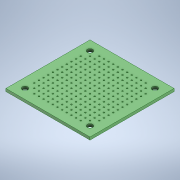
# Autodesk Inventor part: PCB
Saved by Autodesk Inventor 2020.5 (Build 245400000, 400)
## iProperties
Created: 2022-12-14
Part Number: PCB
Material: Generic
Document SubType Name: Modeling
Designer: aivel
Density: 1 g/cm^3
Appearance: Smooth - Dark Forest Green
Author: aivel
Autodesk Inventor part; units mm, degrees
ref_plane "YZ Plane" through (0, 0, 0) normal (1, 0, 0) x (0, 1, 0)
ref_plane "XZ Plane" through (0, 0, 0) normal (0, 1, 0) x (-1, 0, 0)
ref_plane "XY Plane" through (0, 0, 0) normal (0, 0, 1) x (1, 0, 0)
sketch "Sketch1" plane through (0, 0, 0) normal (0, 1, 0) x (-1, 0, 0)
  line L0 (0, 0) -> (-46, 0)
  line L1 (-46, 0) -> (-46, -46)
  line L2 (-46, -46) -> (0, -46)
  line L3 (0, -46) -> (0, 0)
  circle A0 centre (-23, -23) radius 0.375
  line L4 (-23, -46) -> (-23, 0) construction
  line L5 (-46, -23) -> (0, -23) construction
  circle A1 centre (-25.54, -23) radius 0.375
  circle A2 centre (-28.08, -23) radius 0.375
  circle A3 centre (-30.62, -23) radius 0.375
  circle A4 centre (-33.16, -23) radius 0.375
  circle A5 centre (-35.7, -23) radius 0.375
  circle A6 centre (-38.24, -23) radius 0.375
  circle A7 centre (-40.78, -23) radius 0.375
  circle A8 centre (-23, -20.46) radius 0.375
  circle A9 centre (-23, -17.92) radius 0.375
  circle A10 centre (-23, -15.38) radius 0.375
  circle A11 centre (-23, -12.84) radius 0.375
  circle A12 centre (-23, -10.3) radius 0.375
  circle A13 centre (-23, -7.76) radius 0.375
  circle A14 centre (-23, -5.22) radius 0.375
  circle A15 centre (-20.46, -20.46) radius 0.375
  circle A16 centre (-20.46, -17.92) radius 0.375
  circle A17 centre (-20.46, -15.38) radius 0.375
  circle A18 centre (-20.46, -12.84) radius 0.375
  circle A19 centre (-20.46, -10.3) radius 0.375
  circle A20 centre (-20.46, -7.76) radius 0.375
  circle A21 centre (-20.46, -5.22) radius 0.375
  circle A22 centre (-17.92, -20.46) radius 0.375
  circle A23 centre (-17.92, -17.92) radius 0.375
  circle A24 centre (-17.92, -15.38) radius 0.375
  circle A25 centre (-17.92, -12.84) radius 0.375
  circle A26 centre (-17.92, -10.3) radius 0.375
  circle A27 centre (-17.92, -7.76) radius 0.375
  circle A28 centre (-17.92, -5.22) radius 0.375
  circle A29 centre (-15.38, -20.46) radius 0.375
  circle A30 centre (-15.38, -17.92) radius 0.375
  circle A31 centre (-15.38, -15.38) radius 0.375
  circle A32 centre (-15.38, -12.84) radius 0.375
  circle A33 centre (-15.38, -10.3) radius 0.375
  circle A34 centre (-15.38, -7.76) radius 0.375
  circle A35 centre (-15.38, -5.22) radius 0.375
  circle A36 centre (-12.84, -20.46) radius 0.375
  circle A37 centre (-12.84, -17.92) radius 0.375
  circle A38 centre (-12.84, -15.38) radius 0.375
  circle A39 centre (-12.84, -12.84) radius 0.375
  circle A40 centre (-12.84, -10.3) radius 0.375
  circle A41 centre (-12.84, -7.76) radius 0.375
  circle A42 centre (-12.84, -5.22) radius 0.375
  circle A43 centre (-10.3, -20.46) radius 0.375
  circle A44 centre (-10.3, -17.92) radius 0.375
  circle A45 centre (-10.3, -15.38) radius 0.375
  circle A46 centre (-10.3, -12.84) radius 0.375
  circle A47 centre (-10.3, -10.3) radius 0.375
  circle A48 centre (-10.3, -7.76) radius 0.375
  circle A49 centre (-10.3, -5.22) radius 0.375
  circle A50 centre (-7.76, -20.46) radius 0.375
  circle A51 centre (-7.76, -17.92) radius 0.375
  circle A52 centre (-7.76, -15.38) radius 0.375
  circle A53 centre (-7.76, -12.84) radius 0.375
  circle A54 centre (-7.76, -10.3) radius 0.375
  circle A55 centre (-7.76, -7.76) radius 0.375
  circle A56 centre (-5.22, -20.46) radius 0.375
  circle A57 centre (-5.22, -17.92) radius 0.375
  circle A58 centre (-5.22, -15.38) radius 0.375
  circle A59 centre (-5.22, -12.84) radius 0.375
  circle A60 centre (-5.22, -10.3) radius 0.375
  circle A61 centre (-35.7, -23) radius 0.375
  circle A62 centre (-33.16, -23) radius 0.375
  circle A63 centre (-35.7, -20.46) radius 0.375
  circle A64 centre (-33.16, -20.46) radius 0.375
  circle A65 centre (-30.62, -23) radius 0.375
  circle A66 centre (-35.7, -17.92) radius 0.375
  circle A67 centre (-30.62, -17.92) radius 0.375
  circle A68 centre (-28.08, -23) radius 0.375
  circle A69 centre (-25.54, -20.46) radius 0.375
  circle A70 centre (-25.54, -17.92) radius 0.375
  circle A71 centre (-23, -20.46) radius 0.375
  circle A72 centre (-23, -17.92) radius 0.375
  circle A73 centre (-23, -15.38) radius 0.375
  circle A74 centre (-28.08, -17.92) radius 0.375
  circle A75 centre (-30.62, -20.46) radius 0.375
  circle A76 centre (-25.54, -23) radius 0.375
  circle A77 centre (-28.08, -20.46) radius 0.375
  circle A78 centre (-23, -12.84) radius 0.375
  circle A79 centre (-23, -10.3) radius 0.375
  circle A80 centre (-30.62, -15.38) radius 0.375
  circle A81 centre (-23, -7.76) radius 0.375
  circle A82 centre (-23, -5.22) radius 0.375
  circle A83 centre (-25.54, -15.38) radius 0.375
  circle A84 centre (-28.08, -12.84) radius 0.375
  circle A85 centre (-28.08, -15.38) radius 0.375
  circle A86 centre (-25.54, -12.84) radius 0.375
  circle A87 centre (-30.62, -12.84) radius 0.375
  circle A88 centre (-25.54, -10.3) radius 0.375
  circle A89 centre (-25.54, -7.76) radius 0.375
  circle A90 centre (-25.54, -5.22) radius 0.375
  circle A91 centre (-33.16, -12.84) radius 0.375
  circle A92 centre (-33.16, -17.92) radius 0.375
  circle A93 centre (-35.7, -15.38) radius 0.375
  circle A94 centre (-33.16, -15.38) radius 0.375
  circle A95 centre (-35.7, -12.84) radius 0.375
  circle A96 centre (-28.08, -10.3) radius 0.375
  circle A97 centre (-28.08, -7.76) radius 0.375
  circle A98 centre (-28.08, -5.22) radius 0.375
  circle A99 centre (-30.62, -10.3) radius 0.375
  circle A100 centre (-30.62, -7.76) radius 0.375
  circle A101 centre (-30.62, -5.22) radius 0.375
  circle A102 centre (-35.7, -10.3) radius 0.375
  circle A103 centre (-33.16, -7.76) radius 0.375
  circle A104 centre (-35.7, -7.76) radius 0.375
  circle A105 centre (-33.16, -5.22) radius 0.375
  circle A106 centre (-35.7, -5.22) radius 0.375
  circle A107 centre (-33.16, -10.3) radius 0.375
  circle A108 centre (-38.24, -12.84) radius 0.375
  circle A109 centre (-40.78, -12.84) radius 0.375
  circle A110 centre (-40.78, -10.3) radius 0.375
  circle A111 centre (-38.24, -7.76) radius 0.375
  circle A112 centre (-38.24, -10.3) radius 0.375
  circle A113 centre (-38.24, -15.38) radius 0.375
  circle A114 centre (-40.78, -15.38) radius 0.375
  circle A115 centre (-38.24, -17.92) radius 0.375
  circle A116 centre (-40.78, -17.92) radius 0.375
  circle A117 centre (-38.24, -20.46) radius 0.375
  circle A118 centre (-40.78, -20.46) radius 0.375
  circle A119 centre (-38.24, -23) radius 0.375
  circle A120 centre (-40.78, -23) radius 0.375
  circle A121 centre (-10.3, -23) radius 0.375
  circle A122 centre (-12.84, -23) radius 0.375
  circle A123 centre (-15.38, -23) radius 0.375
  circle A124 centre (-17.92, -23) radius 0.375
  circle A125 centre (-20.46, -23) radius 0.375
  circle A126 centre (-7.76, -23) radius 0.375
  circle A127 centre (-5.22, -23) radius 0.375
  circle A128 centre (-17.92, -23) radius 0.375
  circle A129 centre (-15.38, -23) radius 0.375
  circle A130 centre (-12.84, -23) radius 0.375
  circle A131 centre (-10.3, -23) radius 0.375
  circle A132 centre (-7.76, -23) radius 0.375
  circle A133 centre (-5.22, -23) radius 0.375
  circle A134 centre (-20.46, -23) radius 0.375
  circle A135 centre (-25.54, -38.24) radius 0.375
  circle A136 centre (-23, -38.24) radius 0.375
  circle A137 centre (-23, -38.24) radius 0.375
  circle A138 centre (-25.54, -35.7) radius 0.375
  circle A139 centre (-23, -35.7) radius 0.375
  circle A140 centre (-28.08, -35.7) radius 0.375
  circle A141 centre (-23, -40.78) radius 0.375
  circle A142 centre (-23, -40.78) radius 0.375
  circle A143 centre (-28.08, -40.78) radius 0.375
  circle A144 centre (-23, -35.7) radius 0.375
  circle A145 centre (-25.54, -40.78) radius 0.375
  circle A146 centre (-28.08, -38.24) radius 0.375
  circle A147 centre (-23, -33.16) radius 0.375
  circle A148 centre (-23, -33.16) radius 0.375
  circle A149 centre (-23, -30.62) radius 0.375
  circle A150 centre (-23, -30.62) radius 0.375
  circle A151 centre (-23, -28.08) radius 0.375
  circle A152 centre (-23, -28.08) radius 0.375
  circle A153 centre (-23, -25.54) radius 0.375
  circle A154 centre (-25.54, -33.16) radius 0.375
  circle A155 centre (-25.54, -30.62) radius 0.375
  circle A156 centre (-28.08, -33.16) radius 0.375
  circle A157 centre (-28.08, -30.62) radius 0.375
  circle A158 centre (-30.62, -30.62) radius 0.375
  circle A159 centre (-23, -25.54) radius 0.375
  circle A160 centre (-20.46, -25.54) radius 0.375
  circle A161 centre (-20.46, -28.08) radius 0.375
  circle A162 centre (-28.08, -25.54) radius 0.375
  circle A163 centre (-28.08, -28.08) radius 0.375
  circle A164 centre (-25.54, -28.08) radius 0.375
  circle A165 centre (-20.46, -30.62) radius 0.375
  circle A166 centre (-17.92, -25.54) radius 0.375
  circle A167 centre (-15.38, -25.54) radius 0.375
  circle A168 centre (-12.84, -25.54) radius 0.375
  circle A169 centre (-20.46, -33.16) radius 0.375
  circle A170 centre (-20.46, -35.7) radius 0.375
  circle A171 centre (-20.46, -38.24) radius 0.375
  circle A172 centre (-20.46, -40.78) radius 0.375
  circle A173 centre (-17.92, -33.16) radius 0.375
  circle A174 centre (-17.92, -35.7) radius 0.375
  circle A175 centre (-17.92, -38.24) radius 0.375
  circle A176 centre (-17.92, -40.78) radius 0.375
  circle A177 centre (-15.38, -33.16) radius 0.375
  circle A178 centre (-15.38, -35.7) radius 0.375
  circle A179 centre (-15.38, -38.24) radius 0.375
  circle A180 centre (-15.38, -40.78) radius 0.375
  circle A181 centre (-12.84, -33.16) radius 0.375
  circle A182 centre (-12.84, -38.24) radius 0.375
  circle A183 centre (-12.84, -40.78) radius 0.375
  circle A184 centre (-12.84, -35.7) radius 0.375
  circle A185 centre (-17.92, -28.08) radius 0.375
  circle A186 centre (-17.92, -30.62) radius 0.375
  circle A187 centre (-15.38, -28.08) radius 0.375
  circle A188 centre (-15.38, -30.62) radius 0.375
  circle A189 centre (-12.84, -28.08) radius 0.375
  circle A190 centre (-12.84, -30.62) radius 0.375
  circle A191 centre (-10.3, -25.54) radius 0.375
  circle A192 centre (-10.3, -28.08) radius 0.375
  circle A193 centre (-10.3, -30.62) radius 0.375
  circle A194 centre (-10.3, -35.7) radius 0.375
  circle A195 centre (-10.3, -38.24) radius 0.375
  circle A196 centre (-10.3, -40.78) radius 0.375
  circle A197 centre (-10.3, -33.16) radius 0.375
  circle A198 centre (-7.76, -35.7) radius 0.375
  circle A199 centre (-7.76, -38.24) radius 0.375
  circle A200 centre (-7.76, -33.16) radius 0.375
  circle A201 centre (-5.22, -35.7) radius 0.375
  circle A202 centre (-5.22, -33.16) radius 0.375
  circle A203 centre (-7.76, -30.62) radius 0.375
  circle A204 centre (-5.22, -30.62) radius 0.375
  circle A205 centre (-7.76, -28.08) radius 0.375
  circle A206 centre (-5.22, -28.08) radius 0.375
  circle A207 centre (-7.76, -25.54) radius 0.375
  circle A208 centre (-5.22, -25.54) radius 0.375
  circle A209 centre (-33.16, -30.62) radius 0.375
  circle A210 centre (-35.7, -30.62) radius 0.375
  circle A211 centre (-30.62, -25.54) radius 0.375
  circle A212 centre (-30.62, -28.08) radius 0.375
  circle A213 centre (-33.16, -28.08) radius 0.375
  circle A214 centre (-35.7, -28.08) radius 0.375
  circle A215 centre (-35.7, -25.54) radius 0.375
  circle A216 centre (-33.16, -25.54) radius 0.375
  circle A217 centre (-38.24, -30.62) radius 0.375
  circle A218 centre (-38.24, -28.08) radius 0.375
  circle A219 centre (-38.24, -25.54) radius 0.375
  circle A220 centre (-40.78, -30.62) radius 0.375
  circle A221 centre (-40.78, -28.08) radius 0.375
  circle A222 centre (-40.78, -25.54) radius 0.375
  circle A223 centre (-30.62, -33.16) radius 0.375
  circle A224 centre (-30.62, -35.7) radius 0.375
  circle A225 centre (-30.62, -38.24) radius 0.375
  circle A226 centre (-33.16, -33.16) radius 0.375
  circle A227 centre (-33.16, -35.7) radius 0.375
  circle A228 centre (-33.16, -38.24) radius 0.375
  circle A229 centre (-30.62, -40.78) radius 0.375
  circle A230 centre (-35.7, -35.7) radius 0.375
  circle A231 centre (-33.16, -40.78) radius 0.375
  circle A232 centre (-35.7, -40.78) radius 0.375
  circle A233 centre (-35.7, -38.24) radius 0.375
  circle A234 centre (-35.7, -33.16) radius 0.375
  circle A235 centre (-38.24, -35.7) radius 0.375
  circle A236 centre (-38.24, -33.16) radius 0.375
  circle A237 centre (-40.78, -35.7) radius 0.375
  circle A238 centre (-40.78, -33.16) radius 0.375
  circle A239 centre (-38.24, -38.24) radius 0.375
  circle A240 centre (-25.54, -25.54) radius 0.375
  circle A241 centre (-5.22, -40.78) radius 1.5
  circle A242 centre (-40.78, -40.78) radius 1.5
  circle A243 centre (-5.22, -5.22) radius 1.5
  circle A244 centre (-40.78, -5.22) radius 1.5
  constraints: 245 centre point, 106 symmetric about line, 12 end point, 4 midpoint, 2 parallel, 1 horizontal, 1 perpendicular, 127 other
extrude "Extrusion1" add sketch "Sketch1" along normal blind 1.5
body "Solid1"
